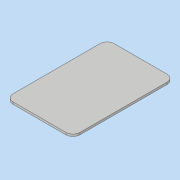
# Autodesk Inventor part: BatteryCaseSide3
Saved by Autodesk Inventor 2017 (Build 210142000, 142)
## iProperties
Created: 2018-02-15
Part Number: BatteryCaseSide3
Material: Generic
Document SubType Name: Modeling
Designer: Derek Wider
Density: 1 g/cm^3
Appearance: Default
Author: Derek Wider
Autodesk Inventor part; units mm, degrees
ref_plane "YZ Plane" through (0, 0, 0) normal (1, 0, 0) x (0, 1, 0)
ref_plane "XZ Plane" through (0, 0, 0) normal (0, 1, 0) x (-1, 0, 0)
ref_plane "XY Plane" through (0, 0, 0) normal (0, 0, 1) x (1, 0, 0)
sketch "Sketch1" plane through (0, 0, 0) normal (0, 1, 0) x (-1, 0, 0)
  line L0 (4.7625, 0) -> (53.0225, 0)
  line L1 (57.785, -4.7625) -> (57.785, -84.1375)
  line L2 (53.0225, -88.9) -> (4.7625, -88.9)
  line L3 (0, -84.1375) -> (0, -4.7625)
  arc A0 (57.785, -4.7625) -> (53.0225, 0) centre (53.0225, -4.7625) ccw
  arc A1 (4.7625, 0) -> (0, -4.7625) centre (4.7625, -4.7625) ccw
  arc A2 (0, -84.1375) -> (4.7625, -88.9) centre (4.7625, -84.1375) ccw
  arc A3 (53.0225, -88.9) -> (57.785, -84.1375) centre (53.0225, -84.1375) ccw
  line L4 (56.1975, -84.1375) -> (56.1975, -4.7625)
  arc A4 (56.1975, -4.7625) -> (53.0225, -1.5875) centre (53.0225, -4.7625) ccw
  line L5 (53.0225, -1.5875) -> (4.7625, -1.5875)
  arc A5 (4.7625, -1.5875) -> (1.5875, -4.7625) centre (4.7625, -4.7625) ccw
  line L6 (1.5875, -4.7625) -> (1.5875, -84.1375)
  arc A6 (1.5875, -84.1375) -> (4.7625, -87.3125) centre (4.7625, -84.1375) ccw
  line L7 (4.7625, -87.3125) -> (53.0225, -87.3125)
  arc A7 (53.0225, -87.3125) -> (56.1975, -84.1375) centre (53.0225, -84.1375) ccw
  line L8 (59.3725, -84.1375) -> (59.3725, -4.7625)
  arc A8 (59.3725, -4.7625) -> (53.0225, 1.5875) centre (53.0225, -4.7625) ccw
  line L9 (53.0225, 1.5875) -> (4.7625, 1.5875)
  arc A9 (4.7625, 1.5875) -> (-1.5875, -4.7625) centre (4.7625, -4.7625) ccw
  line L10 (-1.5875, -4.7625) -> (-1.5875, -84.1375)
  arc A10 (-1.5875, -84.1375) -> (4.7625, -90.4875) centre (4.7625, -84.1375) ccw
  line L11 (4.7625, -90.4875) -> (53.0225, -90.4875)
  arc A11 (53.0225, -90.4875) -> (59.3725, -84.1375) centre (53.0225, -84.1375) ccw
  line L12 (54.2925, -4.7625) -> (54.2925, -84.1375)
  arc A12 (53.0225, -85.4075) -> (54.2925, -84.1375) centre (53.0225, -84.1375) ccw
  line L13 (53.0225, -85.4075) -> (4.7625, -85.4075)
  arc A13 (3.4925, -84.1375) -> (4.7625, -85.4075) centre (4.7625, -84.1375) ccw
  line L14 (3.4925, -84.1375) -> (3.4925, -4.7625)
  arc A14 (4.7625, -3.4925) -> (3.4925, -4.7625) centre (4.7625, -4.7625) ccw
  line L15 (4.7625, -3.4925) -> (53.0225, -3.4925)
  arc A15 (54.2925, -4.7625) -> (53.0225, -3.4925) centre (53.0225, -4.7625) ccw
  line L16 (55.8165, -4.7625) -> (55.8165, -84.1375)
  arc A16 (53.0225, -86.9315) -> (55.8165, -84.1375) centre (53.0225, -84.1375) ccw
  line L17 (53.0225, -86.9315) -> (4.7625, -86.9315)
  arc A17 (1.9685, -84.1375) -> (4.7625, -86.9315) centre (4.7625, -84.1375) ccw
  line L18 (1.9685, -84.1375) -> (1.9685, -4.7625)
  arc A18 (4.7625, -1.9685) -> (1.9685, -4.7625) centre (4.7625, -4.7625) ccw
  line L19 (4.7625, -1.9685) -> (53.0225, -1.9685)
  arc A19 (55.8165, -4.7625) -> (53.0225, -1.9685) centre (53.0225, -4.7625) ccw
  point P0 (0, 0)
  point P1 (0, 0)
  point P2 (57.785, -88.9)
  point P3 (57.785, 0)
  point P4 (0, -88.9)
  dimension "d0" = 88.9
  dimension "d1" = 57.785
  dimension "d2" = 4.7625
  dimension "d3" = 1.5875
  dimension "d4" = 1.5875
  dimension "d5" = 1.905
  dimension "d6" = 0.381
  constraints: 40 end point, 40 point on circle, 20 centre point, 10 parallel, 8 point on line, 8 tangent, 5 perpendicular, 3 equal radius, 1 coincident, 1 horizontal, 28 other
  measures "d0" distance of point (57.785, 0) point (57.785, -88.9)
  measures "d1" distance of point (57.785, -88.9) point (0, -88.9)
  measures "d2" radius of A0
  measures "d3" distance between parallel lines of L1 L4
  measures "d4" distance between parallel lines of L1 L8
  measures "d5" distance between parallel lines of L4 L12
  measures "d6" distance between parallel lines of L4 L16
extrude "Extrusion1" add sketch "Sketch1" along normal blind 1.905 contours L0 A0 L1 A3 L2 A2 L3 A1 | A7 L7 A6 L6 A5 L5 A4 L4 | A11 L11 A10 L10 A9 L9 A8 L8 | L12 A12 L13 A13 L14 A14 L15 A15 | L16 A16 L17 A17 L18 A18 L19 A19
extrude "Extrusion2" add sketch "Sketch1" against normal blind 1.27 contours L16 A16 L17 A17 L18 A18 L19 A19
chamfer "Chamfer1" distance 0.762 angle 45 8 edges at (-28.8925, -1.27, -3.4925) (-3.8645, -1.27, -3.8645) (-3.4925, -1.27, -44.45) (-3.8645, -1.27, -85.0355) (-28.8925, -1.27, -85.4075) (-53.9205, -1.27, -85.0355) (-54.2925, -1.27, -44.45) (-53.9205, -1.27, -3.8645)
equation "\"d3\" = d4"
body "Solid1"
